Autodesk Inventor part; units mm, degrees
(part 3 of 3)
  spline S262 degree 2 poles (-1730.5713, 549.5746) (-1730.5713, 569.7528) (-1742.8484, 590.6605) (-1756.4627, 590.6605) knots 0 0 0 1 2 2 2
  spline S263 degree 2 poles (-1756.4627, 590.6605) (-1764.1207, 590.6605) (-1779.923, 583.3671) (-1786.3654, 577.7755) knots 0 0 0 1 2 2 2
  line L220 (-1786.3654, 577.7755) -> (-1786.3654, 513.2293)
  spline S264 degree 2 poles (-1786.3654, 513.2293) (-1779.1936, 509.7042) (-1768.1321, 506.7869) (-1761.568, 506.7869) knots 0 0 0 1 2 2 2
  spline S265 degree 2 poles (-1761.568, 506.7869) (-1747.1029, 506.7869) (-1730.5713, 527.3298) (-1730.5713, 549.5746) knots 0 0 0 1 2 2 2
  spline S266 degree 2 poles (-1628.5859, 504.842) (-1630.8954, 503.1402) (-1638.675, 497.0624) (-1642.3217, 495.2391) knots 0 0 0 1 2 2 2
  spline S267 degree 2 poles (-1642.3217, 495.2391) (-1647.3055, 492.5648) (-1656.6653, 489.769) (-1665.1742, 489.769) knots 0 0 0 1 2 2 2
  spline S268 degree 2 poles (-1665.1742, 489.769) (-1672.1029, 489.769) (-1684.6231, 494.9959) (-1689.3638, 499.7366) knots 0 0 0 1 2 2 2
  spline S269 degree 2 poles (-1689.3638, 499.7366) (-1693.8614, 504.3558) (-1699.3314, 517.97) (-1699.3314, 525.5065) knots 0 0 0 1 2 2 2
  spline S270 degree 2 poles (-1699.3314, 525.5065) (-1699.3314, 537.1759) (-1689.4854, 553.7075) (-1678.7885, 558.4481) knots 0 0 0 1 2 2 2
  spline S271 degree 2 poles (-1678.7885, 558.4481) (-1669.3071, 562.8242) (-1643.5372, 566.1062) (-1628.5859, 566.9571) knots 0 0 0 1 2 2 2
  line L221 (-1628.5859, 566.9571) -> (-1628.5859, 570.6037)
  spline S272 degree 2 poles (-1628.5859, 570.6037) (-1628.5859, 577.1677) (-1632.5972, 585.312) (-1636.2439, 587.6216) knots 0 0 0 1 2 2 2
  spline S273 degree 2 poles (-1636.2439, 587.6216) (-1639.8906, 589.9311) (-1650.3444, 591.3898) (-1655.9359, 591.3898) knots 0 0 0 1 2 2 2
  spline S274 degree 2 poles (-1655.9359, 591.3898) (-1662.5, 591.3898) (-1680.2471, 587.5) (-1689.1207, 583.7318) knots 0 0 0 1 2 2 2
  line L222 (-1689.1207, 583.7318) -> (-1690.2147, 583.7318)
  line L223 (-1690.2147, 583.7318) -> (-1690.2147, 603.0592)
  spline S275 degree 2 poles (-1690.2147, 603.0592) (-1684.9878, 604.5178) (-1665.4173, 608.1645) (-1655.8144, 608.1645) knots 0 0 0 1 2 2 2
  spline S276 degree 2 poles (-1655.8144, 608.1645) (-1644.145, 608.1645) (-1628.2212, 604.5178) (-1621.9003, 599.7771) knots 0 0 0 1 2 2 2
  spline S277 degree 2 poles (-1621.9003, 599.7771) (-1615.7009, 595.158) (-1609.6231, 580.4498) (-1609.6231, 569.8744) knots 0 0 0 1 2 2 2
  line L224 (-1609.6231, 569.8744) -> (-1609.6231, 492.9295)
  line L225 (-1609.6231, 492.9295) -> (-1628.5859, 492.9295)
  line L226 (-1628.5859, 492.9295) -> (-1628.5859, 504.842)
  line L227 (-1628.5859, 520.6442) -> (-1628.5859, 551.8841)
  spline S278 degree 2 poles (-1628.5859, 551.8841) (-1635.393, 551.2763) (-1655.9359, 549.2099) (-1662.3784, 547.265) knots 0 0 0 1 2 2 2
  spline S279 degree 2 poles (-1662.3784, 547.265) (-1669.9149, 544.9554) (-1679.7609, 535.3525) (-1679.7609, 526.8436) knots 0 0 0 1 2 2 2
  spline S280 degree 2 poles (-1679.7609, 526.8436) (-1679.7609, 517.1191) (-1668.8209, 507.2731) (-1658.3671, 507.2731) knots 0 0 0 1 2 2 2
  spline S281 degree 2 poles (-1658.3671, 507.2731) (-1649.4935, 507.2731) (-1634.9068, 514.9311) (-1628.5859, 520.6442) knots 0 0 0 1 2 2 2
  point P0 (-5000, -2900)
  point P1 (-7550, 741.5985)
  point P2 (-7550, 1200)
  point P3 (-6687.7543, 550)
  point P4 (-9350, 550)
  point P5 (-8412.2457, 550)
  point P6 (-9350, 550)
  point P7 (-7550, 1200)
  point P8 (-2450, 741.5985)
  point P9 (-1273.3317, 550)
  point P10 (-3626.6683, 550)
  point P11 (-2450, 1200)
  point P12 (-4250, 550)
  constraints: 12 midpoint, 3 horizontal alignment, 3 vertical alignment, 1 parallel, 4 other
emboss "Emboss1" sketch "Sketch58" operation cut depth 20 direction (-1, 0, 0) contours S0 S1 L12 L13 L14 S2 S3 | S8 S9 S10 S11 S12 S13 L18 S14 S15 S16 L19 L20 S17 S18 S19 L21 L22 L23 | L25 S24 S25 S26 S27 L26 L27 L28 S28 S29 S30 L29 L30 L31 L32 L33 S31 S32 S33 S34 S35 L34 L35 | S36 S37 L36 L37 S38 S39 S40 L38 L39 L40 L41 L42 | L43 L44 L45 L46 | S41 S42 S43 S44 S45 S46 L47 S47 S48 S49 L48 L49 S50 S51 S52 L50 L51 L52 | L54 L55 S57 S58 S59 L56 L57 L58 L59 L60 S60 S61 L61 | L62 L63 L64 L65 L66 L67 L68 L69 L70 L71 | S62 S63 S64 S65 L72 L73 S66 S67 S68 L74 L75 S69 S70 | L77 L78 L79 L80 | S75 S76 S77 S78 L81 L82 S79 S80 S81 L83 L84 S82 S83 | L86 L87 S88 S89 S90 L88 L89 L90 L91 L92 S91 S92 L93 | S93 S94 L94 L95 L96 L97 L98 S95 S96 | S101 S102 S103 S104 S105 S106 L100 S107 S108 S109 L101 L102 S110 S111 S112 L103 L104 L105 | S117 S118 L107 L108 L109 L110 L111 S119 S120 | S125 S126 S127 S128 S129 S130 L113 S131 S132 S133 L114 L115 S134 S135 S136 L116 L117 L118
emboss "Emboss2" sketch "Sketch58" operation cut depth 20 direction (-1, 0, 0) contours S141 S142 L120 L121 L122 S143 S144 | S149 S150 S151 S152 S153 S154 L126 S155 S156 S157 L127 L128 S158 S159 S160 L129 L130 L131 | L133 S165 S166 S167 S168 L134 L135 L136 S169 S170 S171 L137 L138 L139 L140 L141 S172 S173 S174 S175 S176 L142 L143 | S177 S178 L144 L145 S179 S180 S181 L146 L147 L148 L149 L150 | L151 L152 L153 L154 | S182 S183 S184 S185 S186 S187 L155 S188 S189 S190 L156 L157 S191 S192 S193 L158 L159 L160 | L162 L163 S198 S199 S200 L164 L165 L166 L167 L168 S201 S202 L169 | L170 L171 L172 L173 L174 L175 L176 L177 L178 L179 | S203 S204 S205 S206 L180 L181 S207 S208 S209 L182 L183 S210 S211 | L185 L186 L187 L188 | S216 S217 S218 S219 L189 L190 S220 S221 S222 L191 L192 S223 S224 | L194 L195 S229 S230 S231 L196 L197 L198 L199 L200 S232 S233 L201 | S234 S235 L202 L203 L204 L205 L206 S236 S237 | S242 S243 S244 S245 S246 S247 L208 S248 S249 S250 L209 L210 S251 S252 S253 L211 L212 L213 | S258 S259 L215 L216 L217 L218 L219 S260 S261 | S266 S267 S268 S269 S270 S271 L221 S272 S273 S274 L222 L223 S275 S276 S277 L224 L225 L226
